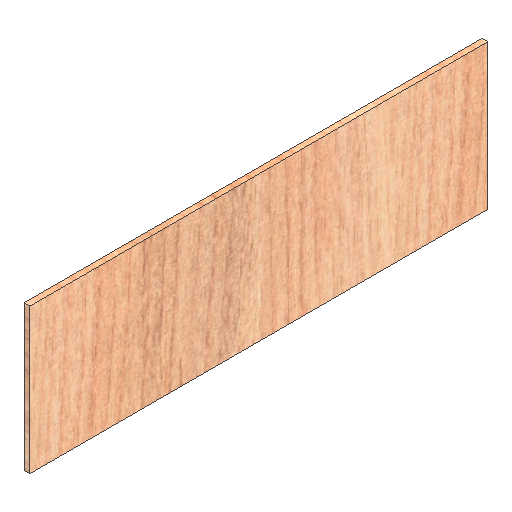
# Autodesk Inventor part: Edge Band - Platform D Flat
Saved by Autodesk Inventor 2021 (Build 250183000, 183)
## iProperties
Created: 2020-05-12
Part Number: Edge Band - Platform D Flat
Material: Wood (Birch)
Document SubType Name: Modeling
Designer: Dan Wikman
Density: 0.55 g/cm^3
Appearance: Birch - Natural Polished
Mass: 69.4606 g
Surface Area: 664.718 cm^2
Volume: 126.292 cm^3
Author: Dan Wikman
Autodesk Inventor part; units mm, degrees
ref_plane "YZ Plane" through (0, 0, 0) normal (1, 0, 0) x (0, 1, 0)
ref_plane "XZ Plane" through (0, 0, 0) normal (0, 1, 0) x (-1, 0, 0)
ref_plane "XY Plane" through (0, 0, 0) normal (0, 0, 1) x (1, 0, 0)
sketch "Sketch1" plane through (0, 0, 0) normal (1, 0, 0) x (0, 1, 0)
  line L0 (62.6437, 125.2128) -> (-37.3563, 125.2128)
  line L1 (-37.3563, 125.2128) -> (-37.3563, -190.5172)
  line L2 (-37.3563, -190.5172) -> (62.6437, -190.5172)
  line L3 (62.6437, -190.5172) -> (62.6437, 125.2128)
  point P0 (0, 0)
  dimension "d0" = 100
  dimension "d1" = 315.73
  constraints: 8 end point, 2 parallel, 1 horizontal, 1 perpendicular
  measures "d0" distance of L1.end L2.end
  measures "d1" distance of L2.end L0.start
extrude "Extrusion1" add sketch "Sketch1" along normal blind 4
body "Solid1"
